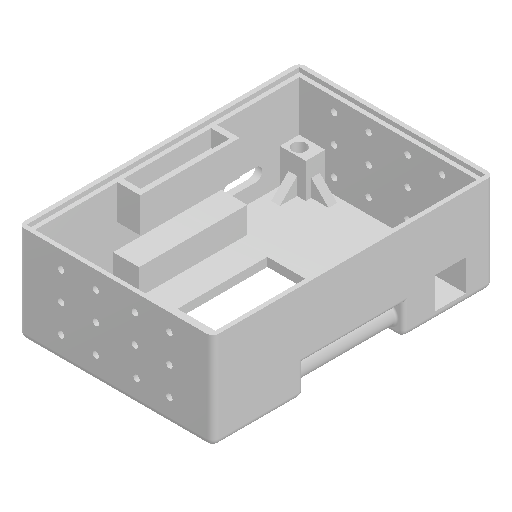
# Autodesk Inventor part: Base
Saved by Autodesk Inventor 2025.2 (Build 292293000, 293)
## iProperties
Created: 2025-10-17
Part Number: Base
Material: ABS Plastic
Document SubType Name: Modeling
Designer: Ricardo
Density: 1.06 g/cm^3
Appearance: Smooth - White
Author: Ricardo
Autodesk Inventor part; units mm, degrees
ref_plane "YZ Plane" through (0, 0, 0) normal (1, 0, 0) x (0, 1, 0)
ref_plane "XZ Plane" through (0, 0, 0) normal (0, 1, 0) x (-1, 0, 0)
ref_plane "XY Plane" through (0, 0, 0) normal (0, 0, 1) x (1, 0, 0)
sketch "Sketch1" plane through (0, 0, 0) normal (0, 1, 0) x (-1, 0, 0)
  line L0 (0, 0) -> (45, 0)
  line L1 (45, 0) -> (45, -65)
  line L2 (45, -65) -> (0, -65)
  line L3 (0, -65) -> (0, 0)
  dimension "d0" = 45
  dimension "d1" = 65
  constraints: 8 end point, 2 parallel, 1 horizontal, 1 perpendicular
  measures "d0" distance of L1.end L2.end
  measures "d1" distance of L0.end L1.end
extrude "Extrusion1" add sketch "Sketch1" against normal blind 3.5
sketch "Sketch2" plane through (0, 0, 0) normal (0, 1, 0) x (1, 0, 0)
  line L0 (-43, 2) -> (-2, 2)
  line L1 (-2, 2) -> (-2, 63)
  line L2 (-2, 63) -> (-43, 63)
  line L3 (-43, 63) -> (-43, 2)
  line L4 (0, 65) -> (-45, 65) projected
  line L5 (-45, 65) -> (-45, 0) projected
  line L6 (-45, 0) -> (0, 0) projected
  line L7 (0, 0) -> (0, 65) projected
  dimension "d4" = 2
  dimension "d5" = 2
  dimension "d6" = 2
  dimension "d7" = 2
  constraints: 8 end point, 2 parallel, 1 horizontal, 1 perpendicular
  measures "d4" distance between parallel lines of L5 L3
  measures "d5" distance between parallel lines of L4 L2
  measures "d6" distance between parallel lines of L7 L1
  measures "d7" distance between parallel lines of L6 L0
extrude "Extrusion2" cut sketch "Sketch2" against normal blind 1.5 contours L3 L2 L1 L0
sketch "Sketch3" plane through (0, -1.5, 0) normal (0, 1, 0) x (1, 0, 0)
  line L0 (-2, 63) -> (-2, 2) projected
  line L1 (-43, 63) -> (-2, 63) projected
  line L2 (-43, 2) -> (-43, 63) projected
  line L3 (-2, 2) -> (-43, 2) projected
  line L4 (-45, 0) -> (0, 0) projected
  line L5 (0, 65) -> (-45, 65) projected
  line L6 (0, 0) -> (0, 65) projected
  line L7 (-45, 65) -> (-45, 0) projected
  line L8 (-30.25, 22.125) -> (-14.75, 22.125)
  line L9 (-14.75, 22.125) -> (-14.75, 42.875)
  line L10 (-14.75, 42.875) -> (-30.25, 42.875)
  line L11 (-30.25, 42.875) -> (-30.25, 22.125)
  line L12 (-43, 2) -> (-43, 63) projected
  line L13 (-22.5, 0) -> (-22.5, 65) construction
  line L14 (0, 32.5) -> (-45, 32.5) construction
  dimension "d10" = 15.5
  dimension "d11" = 20.75
  constraints: 12 end point, 4 midpoint, 3 parallel, 1 horizontal, 1 perpendicular, 2 other
  measures "d10" distance of L10.end L9.end
  measures "d11" distance of L10.end L8.start
extrude "Extrusion3" cut sketch "Sketch3" against normal blind 3 contours L11 L10 L9 L8
sketch "Sketch4" plane through (0, -1.5, 0) normal (0, 1, 0) x (1, 0, 0)
  line L0 (-30.25, 22.125) -> (-30.25, 42.875) construction
  line L1 (-14.75, 42.875) -> (-14.75, 22.125) construction
  line L2 (-14.75, 32.5) -> (-30.25, 32.5) construction
  line L3 (-45, 65) -> (0, 65) construction
  line L4 (-22.5, 65) -> (-22.5, 5) construction
  circle A0 centre (-22.5, 12) radius 5.125
  circle A1 centre (-22.5, 12) radius 6
  line L5 (-45, 0) -> (0, 0) projected
  line L6 (-22.5, 12) -> (-30.82, 16.8036) construction
  line L7 (-22.5, 12) -> (-31.3768, 6.875) construction
  line L8 (-26.9384, 14.5625) -> (-27.9253, 14.5625)
  line L9 (-26.9384, 9.4375) -> (-27.9253, 9.4375)
  point P0 (-28.3926, 10.8696)
  point P1 (-27.5147, 10.9425)
  dimension "d14" = 10.25
  dimension "d15" = 12
  dimension "d181" = 12
  dimension "d200" = 60
  dimension "d201" = 60
  constraints: 12 end point, 6 point on circle, 4 midpoint, 2 centre point, 2 point on line, 1 coincident, 1 horizontal, 1 parallel, 1 vertical
  measures "d14" diameter of A0
  measures "d15" diameter of A1
  measures "d181" distance from line of L5 A0.centre
  measures "d200" angle of L4 L7
  measures "d201" angle of L6 L4
sketch "Sketch6" plane through (0, -1.5, 0) normal (0, 1, 0) x (1, 0, 0)
  line L0 (-14.75, 42.875) -> (-30.25, 42.875) projected
  line L1 (-30.25, 42.875) -> (-30.25, 22.125) projected
  line L2 (-30.25, 22.125) -> (-14.75, 22.125) projected
  line L3 (-14.75, 22.125) -> (-14.75, 42.875) projected
  line L4 (-2, 63) -> (-43, 63) projected
  line L5 (-43, 63) -> (-43, 2) projected
  line L6 (-43, 2) -> (-2, 2) projected
  line L7 (-2, 2) -> (-2, 63) projected
  line L8 (-45, 0) -> (-45, 65) projected
  line L9 (-45, 65) -> (0, 65) projected
  line L10 (0, 65) -> (0, 0) projected
  line L11 (0, 0) -> (-45, 0) projected
  line L12 (-43, 2) -> (-43, 63) projected
  line L13 (-43, 63) -> (-37, 63)
  line L14 (-37, 63) -> (-37, 58.5)
  line L15 (-37, 58.5) -> (-43, 58.5)
  line L16 (-43, 58.5) -> (-43, 63)
  line L17 (-43, 63) -> (-2, 63) projected
  line L18 (-2, 63) -> (-8, 63)
  line L19 (-8, 63) -> (-8, 58.5)
  line L20 (-8, 58.5) -> (-2, 58.5)
  line L21 (-2, 58.5) -> (-2, 63)
  line L22 (-43, 2) -> (-37, 2)
  line L23 (-37, 2) -> (-37, 6.5)
  line L24 (-37, 6.5) -> (-43, 6.5)
  line L25 (-43, 6.5) -> (-43, 2)
  line L26 (-2, 2) -> (-8, 2)
  line L27 (-8, 2) -> (-8, 6.5)
  line L28 (-8, 6.5) -> (-2, 6.5)
  line L29 (-2, 6.5) -> (-2, 2)
  circle A0 centre (-39.5, 4.5) radius 1.6
  circle A1 centre (-5.5, 4.4495) radius 1.4626
  circle A2 centre (-39.5, 60.5) radius 1.6
  circle A3 centre (-5.5, 60.5) radius 1.6
  point P0 (-2, 58.5)
  point P1 (-2, 6.5)
  point P2 (-43, 6.5)
  point P3 (-5, 2)
  dimension "d30" = 6
  dimension "d31" = 4.5
  dimension "d32" = 6
  dimension "d33" = 4.5
  dimension "d34" = 6
  dimension "d35" = 4.5
  dimension "d36" = 6
  dimension "d37" = 4.5
  dimension "d235" = 3.2
  dimension "d236" = 3.5
  dimension "d237" = 2.5
  dimension "d238" = 2.5
  dimension "d239" = 3.5
  dimension "d240" = 3.2
  dimension "d241" = 2.5
  dimension "d242" = 3.5
  dimension "d243" = 3.2
  dimension "d244" = 2.5
  dimension "d245" = 3.5
  constraints: 32 end point, 8 parallel, 4 centre point, 4 horizontal, 4 perpendicular, 1 midpoint
  measures "d30" distance of L14.end L15.end
  measures "d31" distance of L13.end L14.end
  measures "d32" distance of L20.end L19.end
  measures "d33" distance of L18.end L19.end
  measures "d34" distance of L24.end L23.end
  measures "d35" distance of L22.end L23.end
  measures "d36" distance of L27.end L28.end
  measures "d37" distance of L26.end L27.end
  measures "d235" diameter of A0
  measures "d236" distance from line of L5 A0.centre
  measures "d237" distance from line of L6 A0.centre
  measures "d238" distance of point (-5, 2) A1.centre
  measures "d239" distance from line of L7 A1.centre
  measures "d240" diameter of A2
  measures "d241" distance from line of L13 A2.centre
  measures "d242" distance from line of L5 A2.centre
  measures "d243" diameter of A3
  measures "d244" distance from line of L4 A3.centre
  measures "d245" distance from line of L7 A3.centre
extrude "Extrusion6" add sketch "Sketch6" along normal blind 8 contours L7 L20 L19 L4 | L14 L15 L5 L4 | L7 L6 L27 L28 | L24 L23 L6 L5 | A0 | A1 | A2 | A3
sketch "Sketch7" plane through (0, 6.5, 0) normal (0, 1, 0) x (1, 0, 0)
  line L0 (-2, 63) -> (-2, 58.5) projected
  line L1 (-2, 58.5) -> (-8, 58.5) projected
  line L2 (-8, 58.5) -> (-8, 63) projected
  line L3 (-8, 63) -> (-2, 63) projected
  line L4 (-8, 6.5) -> (-2, 6.5) projected
  line L5 (-2, 6.5) -> (-2, 2) projected
  line L6 (-2, 2) -> (-8, 2) projected
  line L7 (-8, 2) -> (-8, 6.5) projected
  line L8 (-37, 58.5) -> (-43, 58.5) projected
  line L9 (-43, 58.5) -> (-43, 63) projected
  line L10 (-43, 63) -> (-37, 63) projected
  line L11 (-37, 63) -> (-37, 58.5) projected
  line L12 (-43, 2) -> (-43, 6.5) projected
  line L13 (-43, 6.5) -> (-37, 6.5) projected
  line L14 (-37, 6.5) -> (-37, 2) projected
  line L15 (-37, 2) -> (-43, 2) projected
  line L16 (-43, 4.25) -> (-40, 4.25) construction
  line L17 (-40.5, 2) -> (-40.5, 4.5) construction
  line L18 (-43, 6.5) -> (-43, 58.5) projected
  line L19 (-2, 58.5) -> (-2, 6.5) projected
  line L20 (0, 0) -> (-45, 0) construction
  line L21 (-22.5, 0) -> (-22.5, 65) construction
  line L22 (-45, 65) -> (0, 65) construction
  circle A0 centre (-40.5, 4.5) radius 1.6
  circle A1 centre (-4.5, 4.5) radius 1.6
  circle A2 centre (-4.5, 60.5) radius 1.6
  circle A3 centre (-40.5, 60.5) radius 1.6
  dimension "d50" = 2.5
  dimension "d51" = 2.5
  dimension "d52" = 2.5
  dimension "d53" = 2.5
  dimension "d54" = 2.5
  dimension "d55" = 2.5
  dimension "d56" = 2.5
  dimension "d228" = 3.2
  dimension "d229" = 2.5
  dimension "d230" = 3.2
  dimension "d231" = 3.2
  dimension "d232" = 3.2
  constraints: 6 end point, 5 coincident, 4 centre point, 3 midpoint, 1 horizontal, 1 perpendicular, 1 point on line
  measures "d50" distance of L17.start L17.end
  measures "d51" distance from line of L5 point (-4.5, 4.5)
  measures "d52" distance from line of L6 point (-4.5, 4.5)
  measures "d53" distance from line of L19 point (-4.5, 60.5)
  measures "d54" distance from line of L3 point (-4.5, 60.5)
  measures "d55" distance from line of L10 point (-40.5, 60.5)
  measures "d56" distance from line of L9 point (-40.5, 60.5)
  measures "d228" diameter of A0
  measures "d229" distance from line of L12 point (-40.5, 4.5)
  measures "d230" diameter of A1
  measures "d231" diameter of A2
  measures "d232" diameter of A3
sketch "Sketch8" plane through (0, 0, 0) normal (0, 1, 0) x (1, 0, 0)
  line L0 (-43, 2) -> (-43, 6.5) projected
  line L1 (-43, 6.5) -> (-37, 6.5) projected
  line L2 (-37, 6.5) -> (-37, 2) projected
  line L3 (-37, 2) -> (-43, 2) projected
  line L4 (-43, 58.5) -> (-43, 6.5) projected
  line L5 (-43, 58.5) -> (-43, 63) projected
  line L6 (-43, 63) -> (-37, 63) projected
  line L7 (-37, 63) -> (-37, 58.5) projected
  line L8 (-37, 2) -> (-8, 2) projected
  line L9 (-2, 2) -> (-8, 2) projected
  line L10 (-2, 6.5) -> (-2, 2) projected
  line L11 (-8, 6.5) -> (-2, 6.5) projected
  line L12 (-8, 2) -> (-8, 6.5) projected
  line L13 (-8, 63) -> (-37, 63) projected
  line L14 (-8, 63) -> (-2, 63) projected
  line L15 (-2, 63) -> (-2, 58.5) projected
  line L16 (-2, 58.5) -> (-8, 58.5) projected
  line L17 (-8, 58.5) -> (-8, 63) projected
  line L18 (-2, 6.5) -> (-2, 58.5) projected
  line L19 (-45, 0) -> (-45, 65) projected
  line L20 (-45, 65) -> (0, 65) projected
  line L21 (0, 65) -> (0, 0) projected
  line L22 (0, 0) -> (-45, 0) projected
  line L23 (-45, 0) -> (0, 0)
  line L24 (0, 0) -> (0, 65)
  line L25 (0, 65) -> (-45, 65)
  line L26 (-45, 65) -> (-45, 0)
  line L27 (-2, 63) -> (-43, 63)
  line L28 (-43, 63) -> (-43, 2)
  line L29 (-43, 2) -> (-2, 2)
  line L30 (-2, 2) -> (-2, 63)
  line L31 (-43, 6.5) -> (-43, 58.5) projected
  line L32 (-45, 65) -> (-45, 0) projected
  line L33 (0, 65) -> (-45, 65) projected
  line L34 (-37, 63) -> (-8, 63) projected
  line L35 (-37, 63) -> (-43, 63) projected
  line L36 (0, 0) -> (0, 65) projected
  line L37 (-2, 58.5) -> (-2, 6.5) projected
  line L38 (-8, 2) -> (-37, 2) projected
  line L39 (-45, 0) -> (0, 0) projected
  line L40 (-43, 2) -> (-2, 2)
  line L41 (-2, 2) -> (-2, 63)
  line L42 (-2, 63) -> (-43, 63)
  line L43 (-43, 63) -> (-43, 2)
  line L44 (0, 0) -> (-45, 0)
  line L45 (-45, 0) -> (-45, 65)
  line L46 (-45, 65) -> (0, 65)
  line L47 (0, 65) -> (0, 0)
  line L48 (-37, 58.5) -> (-43, 58.5) projected
  point P0 (-38.13, 58.5)
  point P1 (-37.5, 3.3857)
  point P2 (-38.5896, 4.5)
  point P3 (-5.5, 3.3968)
  point P4 (-4.3968, 4.5)
  point P5 (-39.1545, 59)
  point P6 (-38, 5.2834)
  point P7 (-38, 59.903)
  point P8 (-2.7165, 59)
  constraints: 32 end point, 8 parallel, 4 horizontal, 4 perpendicular
extrude "Extrusion7" add sketch "Sketch8" along normal blind 18
sketch "Sketch9" plane through (0, 18, 0) normal (0, 1, 0) x (1, 0, 0)
  line L0 (-45, 65) -> (-45, 0) projected
  line L1 (-45, 0) -> (0, 0) projected
  line L2 (0, 0) -> (0, 65) projected
  line L3 (0, 65) -> (-45, 65) projected
  line L4 (-1, 1) -> (-44, 1)
  line L5 (-44, 1) -> (-44, 64)
  line L6 (-44, 64) -> (-1, 64)
  line L7 (-1, 64) -> (-1, 1)
  line L8 (-45, 0) -> (0, 0)
  line L9 (0, 0) -> (0, 65)
  line L10 (0, 65) -> (-45, 65)
  line L11 (-45, 65) -> (-45, 0)
  line L12 (0, 0) -> (-45, 0)
  line L13 (0, 65) -> (0, 0) projected
  line L14 (0, 0) -> (-45, 0) projected
  line L15 (-45, 0) -> (-45, 65) projected
  line L16 (-45, 65) -> (0, 65) projected
  line L17 (-2, 2) -> (-2, 63) projected
  line L18 (-2, 63) -> (-43, 63) projected
  line L19 (-43, 63) -> (-43, 2) projected
  line L20 (-43, 2) -> (-2, 2) projected
  line L21 (-45, 0) -> (0, 0)
  line L22 (0, 0) -> (0, 65)
  line L23 (0, 65) -> (-45, 65)
  line L24 (-45, 65) -> (-45, 0)
  dimension "d57" = 1
  dimension "d58" = 1
  dimension "d59" = 1
  dimension "d60" = 1
  constraints: 26 end point, 7 equal length, 3 horizontal, 3 perpendicular
  measures "d57" distance between parallel lines of L3 L6
  measures "d58" distance between parallel lines of L0 L5
  measures "d59" distance between parallel lines of L1 L4
  measures "d60" distance between parallel lines of L2 L7
extrude "Extrusion8" add sketch "Sketch9" along normal blind 1 contours L3 L2 L1 L0
fillet "Fillet3" radius 1.5 1 edges at (-22.5, -3.5, 0)
fillet "Fillet4" radius 1.5 1 edges at (-22.5, -3.5, -65)
sketch "Sketch10" plane through (-45, 19, -65) normal (-1, 0, 0) x (0, 0, 1)
  line L0 (18, -15.5) -> (12, -15.5) construction
  line L1 (18, -14) -> (12, -14)
  line L2 (12, -17) -> (18, -17)
  arc A0 (18, -17) -> (18, -14) centre (18, -15.5) ccw
  arc A1 (12, -14) -> (12, -17) centre (12, -15.5) ccw
  line L3 (63.5, -22.5) -> (1.5, -22.5) projected
  line L4 (0, -21) -> (0, 0) projected
  point P0 (65, -19)
  point P1 (15, -15.5)
  point P2 (0, -9.5)
  point P3 (0, -6.5)
  dimension "d65" = 6
  dimension "d66" = 3
  dimension "d67" = 5.5
  dimension "d71" = 15
  constraints: 8 end point, 4 point on circle, 4 tangent, 2 centre point, 1 horizontal, 1 midpoint, 1 parallel
  measures "d65" distance of L0.start L0.end
  measures "d66" diameter of A1
  measures "d67" distance between parallel lines of L3 L2
  measures "d71" distance from line of L4 point (15, -15.5)
extrude "Extrusion9" cut sketch "Sketch10" against normal blind 10
sketch "Sketch13" plane through (0, 19, 0) normal (1, 0, 0) x (0, 0, -1)
  line L0 (58.5, -20.5) -> (6.5, -20.5) projected
  line L1 (58.5, -20.5) -> (63, -20.5) projected
  line L2 (63, -20.5) -> (63, -12.5) projected
  line L3 (51.25, -13.25) -> (58.5, -13.25)
  line L4 (58.5, -13.25) -> (58.5, -20.5)
  line L5 (58.5, -20.5) -> (51.25, -20.5)
  line L6 (51.25, -20.5) -> (51.25, -13.25)
  line L7 (51.25, -16.875) -> (58.5, -16.875) construction
  line L8 (54.875, -20.5) -> (54.875, -13.25) construction
  line L9 (65, 0) -> (65, -21) construction
  point P0 (0, -19)
  dimension "d82" = 7.25
  dimension "d83" = 7.25
  dimension "d84" = 0
  dimension "d86" = 6.5
  constraints: 12 end point, 4 midpoint, 2 parallel, 1 horizontal, 1 perpendicular
  measures "d82" distance of L4.end L5.end
  measures "d83" distance of L3.end L4.end
  measures "d84" distance between parallel lines of L0 L5
  measures "d86" distance between parallel lines of L9 L4
extrude "Extrusion11" cut sketch "Sketch13" against normal blind 10
sketch "Sketch17" plane through (0, -1.5, 0) normal (0, 1, 0) x (1, 0, 0)
  line L0 (-8, 45) -> (0, 45)
  line L1 (0, 45) -> (0, 20)
  line L2 (0, 20) -> (-8, 20)
  line L3 (-8, 20) -> (-8, 45)
  line L4 (0, 65) -> (-45, 65) projected
  line L5 (0, 0) -> (0, 65) projected
  line L6 (-22.5, 65) -> (-22.5, 0) construction
  line L7 (0, 0) -> (-45, 0) construction
  line L8 (-37, 45) -> (-45, 45)
  line L9 (-45, 45) -> (-45, 20)
  line L10 (-45, 20) -> (-37, 20)
  line L11 (-37, 20) -> (-37, 45)
  dimension "d104" = 8
  dimension "d105" = 25
  dimension "d106" = 20
  dimension "d107" = 0
  constraints: 18 end point, 4 symmetric about line, 2 midpoint, 2 parallel, 1 horizontal, 1 perpendicular
  measures "d104" distance of L1.end L2.end
  measures "d105" distance of L2.end L0.start
  measures "d106" distance from line of L4 L0.start
  measures "d107" distance between parallel lines of L5 L1
extrude "Extrusion16" add sketch "Sketch17" along normal blind 6
sketch "Sketch19" plane through (-45, 19, -65) normal (-1, 0, 0) x (0, 0, 1)
  arc A0 (18, -17) -> (18, -14) centre (18, -15.5) ccw projected
  line L0 (18, -14) -> (12, -14) projected
  arc A1 (12, -14) -> (12, -17) centre (12, -15.5) ccw projected
  line L1 (12, -17) -> (18, -17) projected
  arc A2 (0, -21) -> (1.5, -22.5) centre (1.5, -21) ccw projected
  line L2 (0, -21) -> (0, 0) projected
  line L3 (0, 0) -> (65, 0) projected
  line L4 (65, 0) -> (65, -21) projected
  arc A3 (63.5, -22.5) -> (65, -21) centre (63.5, -21) ccw projected
  line L5 (63.5, -22.5) -> (1.5, -22.5) projected
  line L6 (45, -14.5) -> (20, -14.5) projected
  line L7 (20, -14.5) -> (20, -20.5) projected
  line L8 (45, -20.5) -> (45, -14.5) projected
  line L9 (21, -22.5) -> (44, -22.5)
  line L10 (44, -22.5) -> (44, -15.5)
  line L11 (44, -15.5) -> (21, -15.5)
  line L12 (21, -15.5) -> (21, -22.5)
  point P0 (65, -19)
  point P1 (19.5, -7.5)
  point P2 (21, -19)
  point P3 (44, -22.5)
  dimension "d110" = 1
  dimension "d111" = 1
  dimension "d112" = 1
  constraints: 8 end point, 2 parallel, 1 horizontal, 1 midpoint, 1 perpendicular, 1 point on line, 3 other
  measures "d110" distance between parallel lines of L8 L10
extrude "Extrusion17" cut sketch "Sketch19" against normal blind 7 contours L12 L11 L10 L5
sketch "Sketch20" plane through (-45, -3.5, -21) normal (0, 0, -1) x (-1, 0, 0)
  line L0 (0, 7) -> (0, 0) projected
  line L1 (0, 0) -> (-7, 0) projected
  circle A0 centre (-3.5, 3.5) radius 2
  point P0 (-45, 3.5)
  dimension "d115" = 3.5
  dimension "d116" = 3.5
  dimension "d117" = 4
  constraints: 1 centre point, 1 coincident
  measures "d115" distance from line of L0 point (-3.5, 3.5)
  measures "d116" distance from line of L1 point (-3.5, 3.5)
  measures "d117" diameter of A0
extrude "Extrusion18" add sketch "Sketch20" along normal blind 24
sketch "Sketch21" plane through (0, 19, 0) normal (1, 0, 0) x (0, 0, -1)
  line L0 (58.5, -20.5) -> (58.5, -13.25) projected
  line L1 (58.5, -13.25) -> (51.25, -13.25) projected
  line L2 (51.25, -13.25) -> (51.25, -20.5) projected
  line L3 (51.25, -20.5) -> (58.5, -20.5) projected
  line L4 (0, 0) -> (65, 0) projected
  line L5 (65, 0) -> (65, -21) projected
  arc A0 (63.5, -22.5) -> (65, -21) centre (63.5, -21) ccw projected
  line L6 (63.5, -22.5) -> (1.5, -22.5) projected
  arc A1 (0, -21) -> (1.5, -22.5) centre (1.5, -21) ccw projected
  line L7 (0, -21) -> (0, 0) projected
  line L8 (44, -15.5) -> (21, -15.5) projected
  line L9 (44, -22.5) -> (44, -15.5) projected
  line L10 (21, -15.5) -> (21, -22.5) projected
  line L11 (21, -22.5) -> (44, -22.5)
  line L12 (44, -22.5) -> (44, -15.5)
  line L13 (44, -15.5) -> (21, -15.5)
  line L14 (21, -15.5) -> (21, -22.5)
  point P0 (0, -19)
  constraints: 8 end point, 2 parallel, 1 horizontal, 1 perpendicular
extrude "Extrusion20" cut sketch "Sketch21" against normal blind 7 contours L10 L8 L9 L6
sketch "Sketch22" plane through (0, -3.5, -44) normal (0, 0, 1) x (1, 0, 0)
  line L0 (0, 7) -> (0, 0) projected
  line L1 (0, 0) -> (-7, 0) projected
  circle A0 centre (-3.5, 3.5) radius 2
  point P0 (0, 3.5)
  dimension "d124" = 3.5
  dimension "d125" = 3.5
  dimension "d126" = 4
  constraints: 1 centre point, 1 coincident
  measures "d124" distance from line of L0 point (-3.5, 3.5)
  measures "d125" distance from line of L1 point (-3.5, 3.5)
  measures "d126" diameter of A0
extrude "Extrusion21" add sketch "Sketch22" along normal blind 24
fillet "Fillet6" radius 1.5 3 edges at (0, -3.0607, -0.4393) (0, 8.5, 0) (0, -3.5, -11.25)
fillet "Fillet9" radius 1 3 edges at (-0.4393, -3.0607, -21) (-4.25, -3.5, -21) (0, 0.75, -21)
fillet "Fillet11" radius 1.5 3 edges at (0, -3.0607, -64.5607) (0, 8.5, -65) (0, -3.5, -53.75)
fillet "Fillet12" radius 1.5 2 edges at (-7, -3.5, -32.5) (-7, -3.5, -20.5)
fillet "Fillet13" radius 1 3 edges at (-0.4393, -3.0607, -44) (0, 0.75, -44) (-5, -3.5, -44)
fillet "Fillet14" radius 1 2 edges at (0, 3.5, -44.5) (0, 3.5, -32)
fillet "Fillet15" radius 1.5 3 edges at (-45, -3.0607, -64.5607) (-45, -3.5, -53.75) (-45, 8.5, -65)
fillet "Fillet16" radius 1.5 3 edges at (-45, -3.0607, -0.4393) (-45, 8.5, 0) (-45, -3.5, -11.25)
sketch "Sketch23" plane through (-43, -1.5, -58.5) normal (1, 0, 0) x (0, 0, -1)
  line L0 (-37.5, 19.5) -> (-14.5, 19.5)
  line L1 (-14.5, 19.5) -> (-14.5, 11.5)
  line L2 (-14.5, 11.5) -> (-37.5, 11.5)
  line L3 (-37.5, 11.5) -> (-37.5, 19.5)
  line L4 (-56.5, 19.5) -> (4.5, 19.5) projected
  line L5 (4.5, 8) -> (4.5, 19.5) projected
  point P0 (-58.5, 1.5)
  dimension "d141" = 23
  dimension "d151" = 8
  dimension "d246" = 19
  constraints: 8 end point, 2 parallel, 1 horizontal, 1 perpendicular, 1 point on line
  measures "d141" distance of L1.end L2.end
  measures "d151" distance of L0.end L1.end
  measures "d246" distance between parallel lines of L1 L5
sketch "Sketch25" plane through (-8, -1.5, -63) normal (-1, 0, 0) x (0, 0, 1)
  line L0 (0, 8) -> (4.5, 8) projected
  line L1 (4.5, 0) -> (4.5, 8) projected
  line L2 (4.5, 0) -> (0, 0) projected
  line L3 (1.25, 0) -> (3.25, 0)
  line L4 (3.25, 0) -> (3.25, 4)
  line L5 (3.25, 4) -> (1.25, 4)
  line L6 (1.25, 4) -> (1.25, 0)
  point P0 (63, 1.5)
  dimension "d157" = 2
  dimension "d158" = 1.25
  dimension "d159" = 4
  constraints: 8 end point, 2 parallel, 1 horizontal, 1 perpendicular, 1 point on line
  measures "d157" distance of L5.end L4.end
  measures "d158" distance between parallel lines of L1 L4
  measures "d159" distance of L3.end L4.end
extrude "Extrusion26" add sketch "Sketch25" along normal blind 4
sketch "Sketch26" plane through (-8, -1.5, -59.75) normal (0, 0, 1) x (1, 0, 0)
  line L0 (0, 4) -> (0, 0) construction
  line L1 (0, 4) -> (-4, 4) construction
  line L2 (-4, 0) -> (-4, 4) construction
  line L3 (0, 0) -> (-4, 0) construction
  line L4 (-4, 0) -> (0, 0) construction
  line L5 (0, 4) -> (-4, 0) construction
  line L6 (-4, 0) -> (0, 4)
  line L7 (-4, 0) -> (-4, 4) projected
  line L8 (-4, 4) -> (-4, 0)
  line L9 (-4, 0) -> (0, 4)
  line L10 (-4, 4) -> (0, 4)
  point P0 (8, 1.5)
  constraints: 12 end point, 3 collinear, 1 point on line
extrude "Extrusion27" cut sketch "Sketch26" against normal blind 2
sketch "Sketch27" plane through (-37, -1.5, -58.5) normal (1, 0, 0) x (0, 0, -1)
  line L0 (0, 8) -> (4.5, 8) projected
  line L1 (0, 0) -> (0, 8) projected
  line L2 (4.5, 8) -> (4.5, 0) projected
  line L3 (4.5, 0) -> (0, 0) projected
  line L4 (4.5, 8) -> (4.5, 0) projected
  line L5 (0, 8) -> (4.5, 8) projected
  line L6 (0, 0) -> (0, 8) projected
  line L7 (0, 0) -> (0, 8) projected
  line L8 (0, 0) -> (0, 8) projected
  line L9 (0, 0) -> (0, 8) projected
  line L10 (4.5, 0) -> (0, 0) projected
  line L11 (3.25, 0) -> (1.25, 0)
  line L12 (1.25, 0) -> (1.25, 4)
  line L13 (1.25, 4) -> (3.25, 4)
  line L14 (3.25, 4) -> (3.25, 0)
  point P0 (-58.5, 1.5)
  dimension "d164" = 2
  dimension "d165" = 1.25
  dimension "d166" = 4
  constraints: 8 end point, 2 parallel, 1 horizontal, 1 perpendicular, 1 point on line
  measures "d164" distance of L12.end L13.end
  measures "d165" distance between parallel lines of L2 L14
  measures "d166" distance of L11.end L12.end
extrude "Extrusion28" add sketch "Sketch27" along normal blind 4 contours L12 L13 L14 L3
sketch "Sketch28" plane through (-37, -1.5, -59.75) normal (0, 0, 1) x (1, 0, 0)
  line L0 (0, 4) -> (4, 4) projected
  line L1 (4, 4) -> (4, 0) projected
  line L2 (4, 0) -> (0, 0) projected
  line L3 (0, 0) -> (0, 4) projected
  line L4 (0, 4) -> (4, 0)
  line L5 (4, 4) -> (4, 0)
  line L6 (4, 4) -> (0, 4)
  point P0 (37, 1.5)
  constraints: 6 end point, 1 collinear
extrude "Extrusion29" cut sketch "Sketch28" against normal blind 2 contours L0 L1 L4
sketch "Sketch29" plane through (-43, -1.5, -58.5) normal (0, 0, 1) x (1, 0, 0)
  line L0 (6, 0) -> (0, 0) projected
  line L1 (6, 0) -> (6, 8) projected
  line L2 (0, 8) -> (6, 8) projected
  line L3 (0, 0) -> (0, 8) projected
  line L4 (6, 0) -> (0, 0) projected
  line L5 (2, 0) -> (4, 0)
  line L6 (4, 0) -> (4, 4)
  line L7 (4, 4) -> (2, 4)
  line L8 (2, 4) -> (2, 0)
  point P0 (43, 1.5)
  dimension "d171" = 2
  dimension "d172" = 2
  dimension "d173" = 4
  constraints: 8 end point, 2 parallel, 1 horizontal, 1 perpendicular, 1 point on line
  measures "d171" distance of L7.end L6.end
  measures "d172" distance between parallel lines of L1 L6
  measures "d173" distance of L5.end L6.end
extrude "Extrusion30" add sketch "Sketch29" along normal blind 4 contours L0 L8 L7 L6
sketch "Sketch30" plane through (-39, -1.5, -58.5) normal (1, 0, 0) x (0, 0, -1)
  line L0 (0, 4) -> (-4, 4) projected
  line L1 (-4, 0) -> (-4, 4) projected
  line L2 (0, 0) -> (-4, 0) projected
  line L3 (0, 4) -> (0, 0) projected
  line L4 (-4, 0) -> (0, 4)
  line L5 (0, 4) -> (-4, 4)
  line L6 (0, 0) -> (0, 8) projected
  line L7 (-4, 0) -> (-4, 4)
  point P0 (-58.5, 1.5)
  constraints: 6 end point, 1 collinear, 1 perpendicular
extrude "Extrusion31" cut sketch "Sketch30" against normal blind 2 contours L4 L1 L0
sketch "Sketch31" plane through (-2, -1.5, -6.5) normal (0, 0, -1) x (-1, 0, 0)
  line L0 (2, 4) -> (4, 4)
  line L1 (4, 4) -> (4, 0)
  line L2 (4, 0) -> (2, 0)
  line L3 (2, 0) -> (2, 4)
  line L4 (6, 0) -> (6, 8) projected
  line L5 (6, 0) -> (0, 0) projected
  point P0 (-2, 1.5)
  dimension "d178" = 2
  dimension "d179" = 2
  dimension "d180" = 4
  constraints: 8 end point, 2 parallel, 1 horizontal, 1 perpendicular, 1 point on line
  measures "d178" distance of L1.end L2.end
  measures "d179" distance between parallel lines of L4 L1
  measures "d180" distance of L0.end L1.end
extrude "Extrusion32" add sketch "Sketch31" along normal blind 4
sketch "Sketch32" plane through (-6, -1.5, -6.5) normal (-1, 0, 0) x (0, 0, 1)
  line L0 (0, 4) -> (0, 0) projected
  line L1 (0, 4) -> (-4, 4) projected
  line L2 (-4, 0) -> (-4, 4) projected
  line L3 (0, 0) -> (-4, 0) projected
  line L4 (-4, 0) -> (0, 4)
  line L5 (0, 4) -> (-4, 4)
  line L6 (-4, 4) -> (-4, 0)
  point P0 (6.5, 1.5)
  constraints: 6 end point, 2 collinear
extrude "Extrusion33" cut sketch "Sketch32" against normal blind 2 contours L4 L2 L1
sketch "Sketch33" plane through (-8, -1.5, -6.5) normal (-1, 0, 0) x (0, 0, 1)
  line L0 (4.5, 0) -> (0, 0) projected
  line L1 (4.5, 8) -> (4.5, 0) projected
  line L2 (0, 8) -> (4.5, 8) projected
  line L3 (0, 0) -> (0, 8) projected
  line L4 (1.25, 4) -> (3.25, 4)
  line L5 (3.25, 4) -> (3.25, 0)
  line L6 (3.25, 0) -> (1.25, 0)
  line L7 (1.25, 0) -> (1.25, 4)
  point P0 (6.5, 1.5)
  point P1 (2.25, 0)
  point P2 (1.25, 0)
  point P3 (3.25, 0)
  dimension "d186" = 2
  dimension "d187" = 1.25
  dimension "d188" = 4
  constraints: 8 end point, 2 midpoint, 2 parallel, 1 horizontal, 1 perpendicular
  measures "d186" distance of L5.end L6.end
  measures "d187" distance between parallel lines of L3 L7
  measures "d188" distance of L6.end L4.start
extrude "Extrusion34" add sketch "Sketch33" along normal blind 4 contours L0 L7 L4 L5
sketch "Sketch34" plane through (-8, -1.5, -5.25) normal (0, 0, -1) x (-1, 0, 0)
  line L0 (0, 0) -> (0, 4) projected
  line L1 (4, 0) -> (0, 0) projected
  line L2 (4, 4) -> (4, 0) projected
  line L3 (0, 4) -> (4, 4) projected
  line L4 (0, 4) -> (4, 0)
  line L5 (4, 4) -> (4, 0) projected
  line L6 (4, 4) -> (0, 4)
  point P0 (-8, 1.5)
  constraints: 4 end point
extrude "Extrusion35" cut sketch "Sketch34" against normal blind 2 contours L3 L2 L4
sketch "Sketch35" plane through (-37, -1.5, -2) normal (1, 0, 0) x (0, 0, -1)
  line L0 (4.5, 0) -> (0, 0) projected
  line L1 (4.5, 0) -> (4.5, 8) projected
  line L2 (0, 8) -> (4.5, 8) projected
  line L3 (0, 0) -> (0, 8) projected
  line L4 (3.25, 4) -> (1.25, 4)
  line L5 (1.25, 4) -> (1.25, 0)
  line L6 (1.25, 0) -> (3.25, 0)
  line L7 (3.25, 0) -> (3.25, 4)
  line L8 (4.5, 0) -> (0, 0) projected
  point P0 (-2, 1.5)
  point P1 (3.25, 0)
  dimension "d193" = 2
  dimension "d194" = 1.25
  dimension "d195" = 4
  constraints: 8 end point, 2 parallel, 1 horizontal, 1 perpendicular, 1 point on line
  measures "d193" distance of L6.end L5.end
  measures "d194" distance between parallel lines of L1 L7
  measures "d195" distance of L6.end L4.start
extrude "Extrusion36" add sketch "Sketch35" along normal blind 4 contours L0 L5 L4 L7
sketch "Sketch36" plane through (-37, -1.5, -5.25) normal (0, 0, -1) x (-1, 0, 0)
  line L0 (0, 4) -> (0, 0) projected
  line L1 (0, 4) -> (-4, 4) projected
  line L2 (-4, 0) -> (-4, 4) projected
  line L3 (0, 0) -> (-4, 0) projected
  line L4 (0, 4) -> (-4, 4) projected
  line L5 (-4, 0) -> (-4, 4)
  line L6 (-4, 4) -> (-4, 0)
  line L7 (0, 4) -> (-4, 4)
  line L8 (0, 4) -> (-4, 0)
  line L9 (-4, 0) -> (-4, 4) projected
  line L10 (-4, 4) -> (0, 4)
  point P0 (-37, 1.5)
  constraints: 10 end point, 2 perpendicular, 1 vertical
extrude "Extrusion37" cut sketch "Sketch36" against normal blind 2 contours L8 L2 L1
extrude "Extrusion38" add sketch "Sketch4" along normal blind 3 contours A0 L8 A1 L9 picked at (-16.8998, 12.8888)
fillet "Fillet18" radius 0.5 1 edges at (-16.5, -1.5, -12)
sketch "Sketch37" plane through (-1.5, -2, 0) normal (0, 0, 1) x (1, 0, 0)
  line L0 (-43.5, 21) -> (-43.5, 0) projected
  line L1 (1.5, 0) -> (1.5, 21) projected
  line L2 (-42, -1.5) -> (0, -1.5) projected
  arc A0 (0, -1.5) -> (1.5, 0) centre (0, 0) ccw projected
  arc A1 (-43.5, 0) -> (-42, -1.5) centre (-42, 0) ccw projected
  circle A2 centre (-33.5, 17) radius 0.75
  circle A3 centre (-33.5, 4) radius 0.75
  circle A4 centre (-33.5, 10.5) radius 0.75
  line L3 (-42, 21) -> (0, 21) projected
  circle A5 centre (-8.5, 17) radius 0.75
  circle A6 centre (-8.5, 4) radius 0.75
  circle A7 centre (-8.5, 10.5) radius 0.75
  circle A8 centre (-25.5, 17) radius 0.75
  circle A9 centre (-25.5, 10.5) radius 0.75
  circle A10 centre (-25.5, 4) radius 0.75
  circle A11 centre (-16.5, 17) radius 0.75
  circle A12 centre (-16.5, 10.5) radius 0.75
  circle A13 centre (-16.0656, 4) radius 0.75
  line L4 (-42, 0) -> (-42, 21) projected
  line L5 (-42, 21) -> (0, 21) projected
  line L6 (0, 21) -> (0, 0) projected
  line L7 (0, 0) -> (-42, 0) projected
  line L8 (-21, 21) -> (-21, 0)
  line L9 (-42, 10.5) -> (0, 10.5)
  point P0 (1.5, 2)
  dimension "d206" = 1.5
  dimension "d207" = 1.5
  dimension "d208" = 1.5
  dimension "d214" = 6.5
  dimension "d259" = 1.5
  dimension "d260" = 1.5
  dimension "d261" = 1.5
  dimension "d263" = 1.5
  dimension "d264" = 1.5
  dimension "d265" = 1.5
  dimension "d266" = 8.5
  dimension "d267" = 8.5
  dimension "d272" = 8
  dimension "d273" = 8
  constraints: 12 centre point, 7 vertical alignment, 4 end point, 4 midpoint, 2 horizontal alignment
  measures "d206" diameter of A2
  measures "d207" diameter of A3
  measures "d208" diameter of A4
  measures "d214" distance of A2.centre A4.centre
  measures "d259" diameter of A8
  measures "d260" diameter of A9
  measures "d261" diameter of A10
  measures "d263" diameter of A11
  measures "d264" diameter of A12
  measures "d265" diameter of A13
  measures "d266" distance from line of L6 A5.centre
  measures "d267" distance from line of L4 A2.centre
  measures "d272" distance of A8.centre A2.centre
  measures "d273" distance of A11.centre A5.centre
extrude "Extrusion39" cut sketch "Sketch37" against normal blind 5 contours A2 | A3 | L9 A4 | A4 L9 | L9 A9 | A9 L9 | L9 A12 | A12 L9 | L9 A7 | A7 L9 | A5 | A6 | A8 | A10 | A11 | A13
sketch "Sketch38" plane through (-1.5, -2, -65) normal (0, 0, -1) x (-1, 0, 0)
  line L0 (0, 21) -> (42, 21) projected
  line L1 (42, 0) -> (42, 21) projected
  line L2 (42, 0) -> (0, 0) projected
  line L3 (0, 0) -> (0, 21) projected
  line L4 (0, 21) -> (42, 21) projected
  line L5 (42, 0) -> (42, 21) projected
  line L6 (42, 0) -> (0, 0) projected
  line L7 (0, 0) -> (0, 21) projected
  circle A0 centre (33.5, 4) radius 0.75 projected
  circle A1 centre (8.5, 17) radius 0.75 projected
  circle A2 centre (8.5, 10.5) radius 0.75 projected
  circle A3 centre (33.5, 10.5) radius 0.75 projected
  circle A4 centre (8.5, 4) radius 0.75 projected
  circle A5 centre (33.5, 17) radius 0.75 projected
  line L8 (6.5, 8.5) -> (6.5, 0.5) projected
  line L9 (6.5, 0.5) -> (35.5, 0.5) projected
  line L10 (35.5, 0.5) -> (35.5, 8.5) projected
  line L11 (41.5, 8.5) -> (35.5, 8.5) projected
  line L12 (41.5, 8.5) -> (41.5, 20) projected
  line L13 (0.5, 20) -> (41.5, 20) projected
  line L14 (0.5, 8.5) -> (0.5, 20) projected
  line L15 (6.5, 8.5) -> (0.5, 8.5) projected
  line L16 (-1.5, 21) -> (-1.5, 0) projected
  line L17 (43.5, 0) -> (43.5, 21) projected
  line L18 (0, -1.5) -> (42, -1.5) projected
  line L19 (0, 21) -> (42, 21) projected
  circle A6 centre (8.5, 17) radius 0.75
  circle A7 centre (8.5, 10.5) radius 0.75
  circle A8 centre (8.5, 4) radius 0.75
  line L20 (28.75, -1.5) -> (13.25, -1.5) construction
  line L21 (21, -1.5) -> (21, 21) construction
  circle A9 centre (33.5, 17) radius 0.75
  circle A10 centre (33.5, 10.5) radius 0.75
  circle A11 centre (33.5, 4) radius 0.75
  circle A12 centre (16.5, 17) radius 0.75
  circle A13 centre (16.5, 10.5) radius 0.75
  circle A14 centre (16.5, 4) radius 0.75
  circle A15 centre (25.5, 17) radius 0.75 projected
  circle A16 centre (25.5, 17) radius 0.75
  circle A17 centre (25.5, 10.5) radius 0.75 projected
  circle A18 centre (25.5, 10.5) radius 0.75
  circle A19 centre (25.5, 4) radius 0.75 projected
  circle A20 centre (25.5, 4) radius 0.75
  point P0 (-1.5, 2)
  dimension "d274" = 1.5
  dimension "d275" = 1.5
  dimension "d276" = 1.5
  dimension "d277" = 8.5
  dimension "d278" = 8
  constraints: 12 centre point, 6 coincident, 3 symmetric about line, 2 concentric, 2 end point, 2 midpoint, 2 vertical alignment, 3 other
  measures "d274" diameter of A12
  measures "d275" diameter of A13
  measures "d276" diameter of A14
  measures "d277" distance from line of L3 A1.centre
  measures "d278" distance of A12.centre A1.centre
extrude "Extrusion40" cut sketch "Sketch38" against normal blind 2 contours A0 | A1 | A2 | A3 | A4 | A5 | A12 | A13 | A14 | A15 | A17 | A19
sketch "Sketch42" plane through (-43, -1.5, -6.5) normal (1, 0, 0) x (0, 0, -1)
  line L0 (40.5, 6.5) -> (46.5, 6.5) projected
  line L1 (46.5, 3.5) -> (40.5, 3.5) projected
  arc A0 (40.5, 6.5) -> (40.5, 3.5) centre (40.5, 5) ccw projected
  line L2 (46.5, 3.5) -> (40.5, 3.5) projected
  arc A1 (40.5, 6.5) -> (40.5, 3.5) centre (40.5, 5) ccw projected
  line L3 (40.5, 6.5) -> (46.5, 6.5) projected
  arc A2 (46.5, 3.5) -> (46.5, 6.5) centre (46.5, 5) ccw projected
  line L4 (-4.5, 19.5) -> (56.5, 19.5) projected
  line L5 (-4.5, 8) -> (-4.5, 19.5) projected
  line L6 (0, 8) -> (-4.5, 8) projected
  line L7 (0, 8) -> (0, 0) projected
  line L8 (0, 0) -> (13.5, 0) projected
  line L9 (13.5, 0) -> (13.5, 6) projected
  line L10 (13.5, 6) -> (38.5, 6) projected
  line L11 (38.5, 6) -> (38.5, 0) projected
  line L12 (38.5, 0) -> (52, 0) projected
  line L13 (52, 0) -> (52, 8) projected
  line L14 (56.5, 8) -> (52, 8) projected
  line L15 (56.5, 8) -> (56.5, 19.5) projected
  line L16 (40.5, 5) -> (46.5, 5) construction
  line L17 (40.5, 3.5) -> (46.5, 3.5)
  line L18 (46.5, 6.5) -> (40.5, 6.5)
  arc A3 (40.5, 6.5) -> (40.5, 3.5) centre (40.5, 5) ccw
  arc A4 (46.5, 3.5) -> (46.5, 6.5) centre (46.5, 5) ccw
  point P0 (-6.5, 1.5)
  point P1 (43.5, 5)
  constraints: 8 end point, 4 point on circle, 4 tangent, 2 centre point, 1 concentric, 1 horizontal, 1 midpoint, 1 parallel
extrude "Extrusion41" cut sketch "Sketch42" against normal blind 10 draft 14 contours L0 A2 L1 A0
fillet "Fillet19" radius 0.5 1 edges at (-39.5, 0, -21)
fillet "Fillet20" radius 0.5 1 edges at (-39.5, 0, -44)
fillet "Fillet21" radius 0.5 1 edges at (-5.5, 0, -21)
fillet "Fillet22" radius 0.5 1 edges at (-5.5, 0, -44)
extrude "Extrusion42" cut sketch "Sketch7" against normal blind 5 contours A0 | A1 | A2 | A3
extrude "Extrusion43" add sketch "Sketch23" along normal blind 5.25
sketch "Sketch44" plane through (0, 18, 0) normal (0, 1, 0) x (1, 0, 0)
  arc A0 (-43.5, 65) -> (-45, 63.5) centre (-43.5, 63.5) ccw projected
  line L0 (-43.5, 65) -> (-1.5, 65) projected
  arc A1 (0, 63.5) -> (-1.5, 65) centre (-1.5, 63.5) ccw projected
  line L1 (0, 63.5) -> (0, 1.5) projected
  arc A2 (-1.5, 0) -> (0, 1.5) centre (-1.5, 1.5) ccw projected
  line L2 (-1.5, 0) -> (-43.5, 0) projected
  arc A3 (-45, 1.5) -> (-43.5, 0) centre (-43.5, 1.5) ccw projected
  line L3 (-45, 1.5) -> (-45, 63.5) projected
  line L4 (-2, 2) -> (-2, 63) projected
  line L5 (-2, 63) -> (-43, 63) projected
  line L6 (-43, 63) -> (-43, 44) projected
  line L7 (-43, 44) -> (-37.75, 44) projected
  line L8 (-37.75, 44) -> (-37.75, 21) projected
  line L9 (-37.75, 21) -> (-43, 21) projected
  line L10 (-43, 21) -> (-43, 2) projected
  line L11 (-43, 2) -> (-2, 2) projected
  line L12 (-1, 1) -> (-1, 64) projected
  line L13 (-1, 64) -> (-44, 64) projected
  line L14 (-44, 64) -> (-44, 1) projected
  line L15 (-43, 22.375) -> (-38.75, 22.375)
  line L16 (-38.75, 22.375) -> (-38.75, 42.625)
  line L17 (-38.75, 42.625) -> (-43, 42.625)
  line L18 (-43, 42.625) -> (-43, 22.375)
  line L19 (-43, 20) -> (-43, 45) construction
  line L20 (-38.75, 32.5) -> (-43, 32.5) construction
  line L21 (-44, 1) -> (-1, 1) projected
  point P0 (0, 0)
  point P1 (-40.875, 42.625)
  dimension "d250" = 1
  dimension "d252" = 0
  dimension "d255" = 20.25
  dimension "d256" = 11.5
  constraints: 10 end point, 3 midpoint, 2 parallel, 2 perpendicular, 1 horizontal
  measures "d250" distance between parallel lines of L8 L16
  measures "d252" distance between parallel lines of L10 L18
  measures "d255" distance between parallel lines of L17 L15
  measures "d256" distance between parallel lines of L7 L20
extrude "Extrusion44" cut sketch "Sketch44" against normal blind 4 contours L18 L17 L16 L15
body "Solid1"
